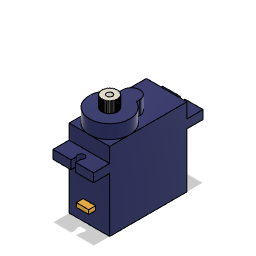
Mechanism v8 v6 (Autodesk Fusion 360 archive; units mm, degrees)
design "servo"
Autodesk Fusion 360 part; units mm, degrees
sketch "Left" plane through (0, 0, 0) normal (1, 0, 0) x (0, 0, -1)
  line L0 (-21.4055, -22.0984) -> (1.0945, -22.0984)
  line L1 (-21.4055, 4.6016) -> (1.0945, 4.6016)
  line L2 (-21.4055, 0.6016) -> (1.0945, 0.6016)
  line L3 (-21.4055, 0.6016) -> (-21.4055, 4.6016)
  line L4 (5.7945, -22.0984) -> (5.7945, -6.1984)
  line L5 (-26.1055, -6.1984) -> (-26.1055, -3.6984)
  line L6 (-26.1055, -3.6984) -> (-21.4055, -3.6984)
  line L7 (1.0945, -3.6984) -> (5.7945, -3.6984)
  line L8 (-26.1055, -6.1984) -> (-21.4055, -6.1984)
  line L9 (1.0945, -6.1984) -> (5.7945, -6.1984)
  line L10 (1.0945, -22.0984) -> (1.0945, -6.1984)
  line L11 (1.0945, -3.6984) -> (1.0945, 0.6016)
  line L12 (-21.4055, -22.0984) -> (-21.4055, -6.1984)
  line L13 (-21.4055, -3.6984) -> (-21.4055, 0.6016)
  line L14 (-15.5055, 0.6016) -> (-15.5055, 13)
  line L15 (-6.7055, 0.6016) -> (-6.7055, 13)
  line L16 (1.0945, -22.0984) -> (1.0945, -6.1984)
  line L17 (1.0945, -3.6984) -> (1.0945, 13)
  line L18 (5.7945, -3.6984) -> (5.7945, -6.1984)
  dimension "d1" = 22.5
  dimension "d2" = 26.7
  dimension "d3" = 22.7
  dimension "d4" = 4
  dimension "d5" = 22.7
  dimension "d13" = 5.9
  constraint perpendicular L1 L3
  constraint parallel L0 L6
  constraint parallel L0 L8
  constraint parallel L5 L12
  constraint coincident L6.end L12
  constraint coincident L7.start L10
  constraint collinear L6 L7
  constraint collinear L8 L9
  constraint parallel L4 L10
  constraint collinear L10 L11
  constraint collinear L12 L13
  constraint parallel L3 L14
  constraint parallel L14 L16
  constraint collinear L16 L17
  constraint parallel L14 L15
  constraint coincident L2 L15.start
  constraint coincident L2 L14.start
  constraint perpendicular L9 L18
  measures "d1" distance of L0.start L0.end
  measures "d4" distance of L1.start L2.start
  measures "d5" distance of L0.start L2.start
  measures "d13" distance of L3 L14
extrude "Extrude1" add sketch "Left" along normal mid plane 11.8 contours L0 L2 L5 L6 L7 L8 L9 L10 L11 L12 L13 L16 L17 L18 makes body 1
sketch "TOP" plane through (0, 0.6016, 0) normal (0, 1, 0) x (-1, 0, 0)
  line L0 (5.9, 21.4055) -> (-5.9, 21.4055)
  line L1 (-5.9, 21.4055) -> (-5.9, -1.0945)
  line L2 (-5.9, -1.0945) -> (5.9, -1.0945)
  line L3 (5.9, -1.0945) -> (5.9, 21.4055)
  circle A0 centre (0, 15.5055) radius 2.3
  circle A1 centre (0, 15.5055) radius 0.85
  line L4 (0, -1.0945) -> (0, 27)
  line L5 (0, 27) -> (0, -1.0945)
  arc A2 (-2.5, 9.2055) -> (2.5, 9.2055) centre (0, 9.2055) ccw
  line L6 (-2.5, 9.2055) -> (-2.5, 10.1613)
  line L7 (2.5, 9.2055) -> (2.5, 10.1613)
  arc A3 (2.5, 10.1613) -> (-2.5, 10.1613) centre (0, 15.5055) ccw
  line L8 (5.9, -5.7945) -> (-5.9, -5.7945)
  line L9 (-0.65, -4.2545) -> (-0.65, -5.7945)
  line L10 (0.65, -4.2545) -> (0.65, -5.7945)
  arc A4 (0.65, -4.2545) -> (-0.65, -4.2545) centre (0, -3.4945) ccw
  line L11 (5.9, 26.1055) -> (-5.9, 26.1055)
  arc A5 (-0.65, 24.5654) -> (0.65, 24.5654) centre (0, 23.8055) ccw
  line L12 (0.65, 24.5654) -> (0.65, 26.1055)
  line L13 (-0.65, 24.5654) -> (-0.65, 26.1055)
  point P0 (0, 15.5055)
  point P1 (0, 6.7055)
  point P2 (0, -1.0945)
  point P3 (5.9, -5.7945)
  point P4 (-5.9, -5.7945)
  point P5 (0, -5.7945)
  point P6 (5.9, 26.1055)
  point P7 (-5.9, 26.1055)
  point P8 (0, 26.1055)
  point P9 (0, 21.4055)
  dimension "d16" = 4.6
  dimension "d17" = 1.7
  dimension "d18" = 11.8
  dimension "d27" = 2
  dimension "d31" = 2
  constraint coincident P0 A0.centre
  constraint concentric A1 A3
  constraint coincident P1 A2
  constraint coincident P2 L4.start
  constraint perpendicular L0 L4
  constraint parallel L4 L6
  constraint parallel L4 L7
  constraint coincident P3 L8.start
  constraint coincident P4 L8.end
  constraint coincident P6 L11.start
  constraint coincident P7 L11.end
  constraint coincident L11 L12.end
  constraint coincident L11 L13.end
  measures "d16" diameter of A0
  measures "d17" diameter of A1
  measures "d18" diameter of A3
  measures "d27" diameter of A4
  measures "d31" diameter of A5
extrude "Extrude2" add sketch "TOP" along normal blind 4 contours A0 L4 L5 A2 L7 A3 | A0 L4 L5 A2 L6 A3 bodies 1
extrude "Extrude3" add sketch "TOP" along normal blind 7.2 separate body contours A0 A1 L4 L5 | A0 A1 L4 L5 makes body 2
extrude "Extrude4" cut sketch "TOP" against normal through all contours L4 L5 L11 A5 L13 | L4 L5 L11 A5 L12 bodies 1
extrude "Extrude5" cut sketch "TOP" against normal through all contours L8 L9 L10 A4 bodies 1
sketch "Front" plane through (0, 0, 21.4055) normal (0, 0, 1) x (1, 0, 0)
  line L0 (-5.9, -22.0984) -> (5.9, -22.0984)
  line L1 (5.9, -22.0984) -> (5.9, -6.1984)
  line L2 (5.9, -6.1984) -> (-5.9, -6.1984)
  line L3 (-5.9, -6.1984) -> (-5.9, -22.0984)
  line L4 (-1.8, -17.5984) -> (1.8, -17.5984)
  line L5 (0, -22.0984) -> (0, -6.1984)
  line L6 (1.8, -17.5984) -> (1.8, -16.3984)
  line L7 (-1.8, -17.5984) -> (-1.8, -16.3984)
  line L8 (-1.8, -16.3984) -> (1.8, -16.3984)
extrude "Extrude6" add sketch "Front" along normal blind 2 separate body contours L4 L5 L6 L8 | L4 L5 L7 L8 makes body 3
copy_body "Body->Comp1" bodies 3 removing the originals makes body 4 in component "Prikljiček"
copy_body "Body->Comp2" bodies 2 removing the originals makes body 5 in component "OSovina"
copy_body "Body->Comp3" bodies 1 removing the originals makes body 6 in component "Ohisje"
sketch "Sketch1" plane through (0, 7.8016, 0) normal (0, 1, 0) x (-1, 0, 0) in component "OSovina"
  circle A0 centre (0, 15.5055) radius 0.85
  circle A1 centre (0, 15.5055) radius 2.3
  circle A2 centre (0, 15.5055) radius 2.3
  circle A3 centre (-0.0134, 13.2055) radius 0.125
  dimension "d42" = 0.25
  constraint coincident A2 A3.centre
  measures "d42" diameter of A3
extrude "Extrude1'" cut sketch "Sketch1" against normal up to surface (3.2 mm away) contours A1 A2 A3 | A1 A2 A3 picked at (-0.0101, 13.2473) picked at (-0.0141, 13.1641) bodies 5 in component "OSovina"
pattern_circular "C-Pattern1" count 28 over 360 about axis through (0, 15.4797, 15.5055) along (0, -1, 0) of "Extrude1'" in component "OSovina"
component "Prikljiček" placed x (1, 0, 0) y (0, 1, 0) z (0, 0, 1) at (0, 0, 0)
component "OSovina" placed x (1, 0, 0) y (0, 1, 0) z (0, 0, 1) at (0, 0, 0)
component "Ohisje" placed x (1, 0, 0) y (0, 1, 0) z (0, 0, 1) at (0, 0, 0)
